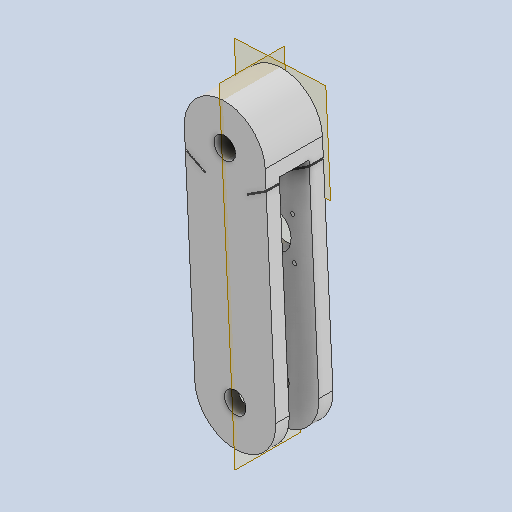
# Autodesk Inventor part: arm segment 2
Saved by Autodesk Inventor 2024 (Build 280153000, 153)
## iProperties
Created: 2024-01-05
Part Number: arm segment 2
Material: Generic
Document SubType Name: Modeling
Designer: MaartenGeorgesBuelen
Density: 1 g/cm^3
Appearance: Default
Author: MaartenGeorgesBuelen
Autodesk Inventor part; units mm, degrees
ref_plane "YZ Plane" through (0, 0, 0) normal (1, 0, 0) x (0, 1, 0)
ref_plane "XZ Plane" through (0, 0, 0) normal (0, 1, 0) x (-1, 0, 0)
ref_plane "Work Plane1" through (-3.789, 77.9897, -50.5078) normal (0, 0, 1) x (0.9988137, 0.0486948, 0)
sketch "Sketch1" plane through (-3.789, 77.9897, -50.5078) normal (0, 0, 1) x (0.9988137, 0.0486948, 0)
  arc A0 (29.7203, 14.7064) -> (-30.2768, 14.1208) centre (-0.263, 12.8566) ccw projected
  circle A1 centre (-0.263, 12.8566) radius 30.0404
  line L0 (25.8606, -3.9877) -> (23.2644, -5.4805)
  line L1 (23.2644, -5.4805) -> (23.0289, -5.0709)
  line L2 (23.0289, -5.0709) -> (23.1978, -4.9738)
  arc A2 (23.1978, -4.9738) -> (23.2457, -4.8334) centre (23.1417, -4.8762) ccw
  arc A3 (23.1909, -4.5987) -> (23.2457, -4.8334) centre (23.9391, -4.5475) ccw
  arc A4 (23.8396, -4.2256) -> (23.1909, -4.5987) centre (23.6062, -4.5703) ccw
  arc A5 (24.0148, -4.3911) -> (23.8396, -4.2256) centre (23.419, -4.8466) ccw
  arc A6 (24.0148, -4.3911) -> (24.1603, -4.4203) centre (24.1042, -4.3228) ccw
  line L3 (24.1603, -4.4203) -> (24.4982, -4.2261)
  arc A7 (24.4982, -4.2261) -> (24.5461, -4.0857) centre (24.4421, -4.1285) ccw
  arc A8 (24.4912, -3.8509) -> (24.5461, -4.0857) centre (25.2395, -3.7998) ccw
  arc A9 (25.1399, -3.4779) -> (24.4912, -3.8509) centre (24.9065, -3.8226) ccw
  arc A10 (25.3152, -3.6434) -> (25.1399, -3.4779) centre (24.7193, -4.0989) ccw
  arc A11 (25.3152, -3.6434) -> (25.4607, -3.6726) centre (25.4046, -3.5751) ccw
  line L4 (25.4607, -3.6726) -> (25.6251, -3.5781)
  line L5 (23.2786, -5.4919) -> (20.6824, -6.9847)
  line L6 (21.5783, -5.9245) -> (21.9162, -5.7302)
  arc A12 (21.9162, -5.7302) -> (21.9641, -5.5898) centre (21.8601, -5.6327) ccw
  arc A13 (21.9092, -5.3551) -> (21.9641, -5.5898) centre (22.6575, -5.304) ccw
  arc A14 (22.5579, -4.9821) -> (21.9092, -5.3551) centre (22.3245, -5.3267) ccw
  arc A15 (22.7332, -5.1476) -> (22.5579, -4.9821) centre (22.1373, -5.6031) ccw
  arc A16 (22.7332, -5.1476) -> (22.8787, -5.1768) centre (22.8226, -5.0793) ccw
  line L7 (22.8787, -5.1768) -> (23.0431, -5.0822)
  line L8 (20.6824, -6.9847) -> (20.4469, -6.5751)
  line L9 (20.4469, -6.5751) -> (20.6158, -6.478)
  arc A17 (21.4328, -5.8953) -> (21.5783, -5.9245) centre (21.5222, -5.827) ccw
  arc A18 (21.4328, -5.8953) -> (21.2576, -5.7298) centre (20.837, -6.3508) ccw
  arc A19 (21.2576, -5.7298) -> (20.6089, -6.1028) centre (21.0242, -6.0744) ccw
  arc A20 (20.6089, -6.1028) -> (20.6637, -6.3375) centre (21.3571, -6.0517) ccw
  arc A21 (20.6158, -6.478) -> (20.6637, -6.3375) centre (20.5597, -6.3804) ccw
  line L10 (20.7516, -6.9254) -> (18.1554, -8.4182)
  line L11 (19.0513, -7.3581) -> (19.3891, -7.1638)
  arc A22 (19.3891, -7.1638) -> (19.4371, -7.0234) centre (19.3331, -7.0663) ccw
  arc A23 (19.3822, -6.7887) -> (19.4371, -7.0234) centre (20.1305, -6.7375) ccw
  arc A24 (20.0309, -6.4156) -> (19.3822, -6.7887) centre (19.7975, -6.7603) ccw
  arc A25 (20.2062, -6.5811) -> (20.0309, -6.4156) centre (19.6103, -7.0366) ccw
  arc A26 (20.2062, -6.5811) -> (20.3516, -6.6103) centre (20.2956, -6.5128) ccw
  line L12 (20.3516, -6.6103) -> (20.5161, -6.5158)
  line L13 (18.1554, -8.4182) -> (17.9199, -8.0086)
  line L14 (17.9199, -8.0086) -> (18.0888, -7.9115)
  arc A27 (18.9058, -7.3289) -> (19.0513, -7.3581) centre (18.9952, -7.2605) ccw
  arc A28 (18.9058, -7.3289) -> (18.7306, -7.1634) centre (18.31, -7.7843) ccw
  arc A29 (18.7306, -7.1634) -> (18.0819, -7.5364) centre (18.4971, -7.508) ccw
  arc A30 (18.0819, -7.5364) -> (18.1367, -7.7711) centre (18.8301, -7.4852) ccw
  arc A31 (18.0888, -7.9115) -> (18.1367, -7.7711) centre (18.0327, -7.814) ccw
  line L15 (18.2037, -8.3904) -> (15.6075, -9.8833)
  line L16 (16.5034, -8.8231) -> (16.8413, -8.6288)
  arc A32 (16.8413, -8.6288) -> (16.8892, -8.4884) centre (16.7852, -8.5313) ccw
  arc A33 (16.8343, -8.2537) -> (16.8892, -8.4884) centre (17.5826, -8.2026) ccw
  arc A34 (17.4831, -7.8807) -> (16.8343, -8.2537) centre (17.2496, -8.2253) ccw
  arc A35 (17.6583, -8.0462) -> (17.4831, -7.8807) centre (17.0625, -8.5016) ccw
  arc A36 (17.6583, -8.0462) -> (17.8038, -8.0754) centre (17.7477, -7.9779) ccw
  line L17 (17.8038, -8.0754) -> (17.9682, -7.9808)
  line L18 (15.6075, -9.8833) -> (15.372, -9.4737)
  line L19 (15.372, -9.4737) -> (15.5409, -9.3765)
  arc A37 (16.358, -8.7939) -> (16.5034, -8.8231) centre (16.4473, -8.7256) ccw
  arc A38 (16.358, -8.7939) -> (16.1827, -8.6284) centre (15.7621, -9.2494) ccw
  arc A39 (16.1827, -8.6284) -> (15.534, -9.0014) centre (15.9493, -8.973) ccw
  arc A40 (15.534, -9.0014) -> (15.5889, -9.2361) centre (16.2822, -8.9503) ccw
  arc A41 (15.5409, -9.3765) -> (15.5889, -9.2361) centre (15.4848, -9.279) ccw
  line L20 (20.5161, -6.5158) -> (20.6588, -6.4337)
  line L21 (20.6506, -6.9835) -> (20.6824, -6.9847)
  line L22 (23.0238, -5.0934) -> (23.0289, -5.0709)
  line L23 (23.2786, -5.4919) -> (23.3153, -5.4513)
  line L24 (-0.263, 12.8566) -> (-0.263, -17.1838)
  line L25 (-26.3867, -3.9877) -> (-23.7905, -5.4805)
  line L26 (-24.6864, -4.4203) -> (-25.0243, -4.2261)
  arc A42 (-25.0722, -4.0857) -> (-25.0243, -4.2261) centre (-24.9682, -4.1285) ccw
  arc A43 (-25.0722, -4.0857) -> (-25.0173, -3.8509) centre (-25.7656, -3.7998) ccw
  arc A44 (-25.0173, -3.8509) -> (-25.666, -3.4779) centre (-25.4326, -3.8226) ccw
  arc A45 (-25.666, -3.4779) -> (-25.8413, -3.6434) centre (-25.2454, -4.0989) ccw
  arc A46 (-25.9867, -3.6726) -> (-25.8413, -3.6434) centre (-25.9307, -3.5751) ccw
  line L27 (-25.9867, -3.6726) -> (-26.1512, -3.5781)
  line L28 (-23.7905, -5.4805) -> (-23.555, -5.0709)
  line L29 (-23.555, -5.0709) -> (-23.7239, -4.9738)
  arc A47 (-24.6864, -4.4203) -> (-24.5409, -4.3911) centre (-24.6303, -4.3228) ccw
  arc A48 (-24.3657, -4.2256) -> (-24.5409, -4.3911) centre (-23.9451, -4.8466) ccw
  arc A49 (-23.717, -4.5987) -> (-24.3657, -4.2256) centre (-24.1322, -4.5703) ccw
  arc A50 (-23.7718, -4.8334) -> (-23.717, -4.5987) centre (-24.4652, -4.5475) ccw
  arc A51 (-23.7718, -4.8334) -> (-23.7239, -4.9738) centre (-23.6678, -4.8762) ccw
  line L30 (-21.2085, -6.9847) -> (-20.973, -6.5751)
  line L31 (-20.973, -6.5751) -> (-21.1419, -6.478)
  arc A52 (-21.1898, -6.3375) -> (-21.1419, -6.478) centre (-21.0858, -6.3804) ccw
  arc A53 (-21.1898, -6.3375) -> (-21.135, -6.1028) centre (-21.8832, -6.0517) ccw
  arc A54 (-22.1044, -5.9245) -> (-21.9589, -5.8953) centre (-22.0483, -5.827) ccw
  arc A55 (-21.135, -6.1028) -> (-21.7837, -5.7298) centre (-21.5502, -6.0744) ccw
  arc A56 (-21.7837, -5.7298) -> (-21.9589, -5.8953) centre (-21.3631, -6.3508) ccw
  line L32 (-23.8047, -5.4919) -> (-21.2085, -6.9847)
  line L33 (-22.1044, -5.9245) -> (-22.4423, -5.7302)
  arc A57 (-22.4902, -5.5898) -> (-22.4423, -5.7302) centre (-22.3862, -5.6327) ccw
  arc A58 (-22.4902, -5.5898) -> (-22.4353, -5.3551) centre (-23.1836, -5.304) ccw
  arc A59 (-22.4353, -5.3551) -> (-23.084, -4.9821) centre (-22.8506, -5.3267) ccw
  arc A60 (-23.4047, -5.1768) -> (-23.2593, -5.1476) centre (-23.3487, -5.0793) ccw
  line L34 (-23.4047, -5.1768) -> (-23.5692, -5.0822)
  arc A61 (-23.084, -4.9821) -> (-23.2593, -5.1476) centre (-22.6634, -5.6031) ccw
  line L35 (-18.6815, -8.4182) -> (-18.4459, -8.0086)
  line L36 (-18.4459, -8.0086) -> (-18.6149, -7.9115)
  arc A62 (-18.6628, -7.7711) -> (-18.6149, -7.9115) centre (-18.5588, -7.814) ccw
  arc A63 (-18.6628, -7.7711) -> (-18.6079, -7.5364) centre (-19.3562, -7.4852) ccw
  arc A64 (-19.5774, -7.3581) -> (-19.4319, -7.3289) centre (-19.5213, -7.2605) ccw
  arc A65 (-18.6079, -7.5364) -> (-19.2567, -7.1634) centre (-19.0232, -7.508) ccw
  arc A66 (-19.2567, -7.1634) -> (-19.4319, -7.3289) centre (-18.836, -7.7843) ccw
  line L37 (-21.2777, -6.9254) -> (-18.6815, -8.4182)
  line L38 (-19.5774, -7.3581) -> (-19.9152, -7.1638)
  arc A67 (-19.9632, -7.0234) -> (-19.9152, -7.1638) centre (-19.8592, -7.0663) ccw
  arc A68 (-19.9632, -7.0234) -> (-19.9083, -6.7887) centre (-20.6565, -6.7375) ccw
  arc A69 (-19.9083, -6.7887) -> (-20.557, -6.4156) centre (-20.3236, -6.7603) ccw
  arc A70 (-20.8777, -6.6103) -> (-20.7323, -6.5811) centre (-20.8216, -6.5128) ccw
  line L39 (-20.8777, -6.6103) -> (-21.0422, -6.5158)
  arc A71 (-20.557, -6.4156) -> (-20.7323, -6.5811) centre (-20.1364, -7.0366) ccw
  line L40 (-16.1336, -9.8833) -> (-15.8981, -9.4737)
  line L41 (-15.8981, -9.4737) -> (-16.067, -9.3765)
  arc A72 (-16.1149, -9.2361) -> (-16.067, -9.3765) centre (-16.0109, -9.279) ccw
  arc A73 (-16.1149, -9.2361) -> (-16.0601, -9.0014) centre (-16.8083, -8.9503) ccw
  arc A74 (-17.0295, -8.8231) -> (-16.884, -8.7939) centre (-16.9734, -8.7256) ccw
  arc A75 (-16.0601, -9.0014) -> (-16.7088, -8.6284) centre (-16.4754, -8.973) ccw
  arc A76 (-16.7088, -8.6284) -> (-16.884, -8.7939) centre (-16.2882, -9.2494) ccw
  line L42 (-18.7298, -8.3904) -> (-16.1336, -9.8833)
  line L43 (-17.0295, -8.8231) -> (-17.3674, -8.6288)
  arc A77 (-17.4153, -8.4884) -> (-17.3674, -8.6288) centre (-17.3113, -8.5313) ccw
  arc A78 (-17.4153, -8.4884) -> (-17.3604, -8.2537) centre (-18.1087, -8.2026) ccw
  arc A79 (-17.3604, -8.2537) -> (-18.0091, -7.8807) centre (-17.7757, -8.2253) ccw
  arc A80 (-18.3299, -8.0754) -> (-18.1844, -8.0462) centre (-18.2738, -7.9779) ccw
  line L44 (-18.3299, -8.0754) -> (-18.4943, -7.9808)
  arc A81 (-18.0091, -7.8807) -> (-18.1844, -8.0462) centre (-17.5885, -8.5016) ccw
  line L45 (-21.0422, -6.5158) -> (-21.1849, -6.4337)
  line L46 (-21.1767, -6.9835) -> (-21.2085, -6.9847)
  line L47 (-23.5499, -5.0934) -> (-23.555, -5.0709)
  line L48 (-23.8047, -5.4919) -> (-23.8414, -5.4513)
  line L49 (-30.3034, 12.8566) -> (29.7773, 12.8566)
  line L50 (29.7773, 12.8566) -> (29.7773, -147.1434)
  line L51 (29.7773, -147.1434) -> (-30.3034, -147.1434)
  line L52 (-30.3034, -147.1434) -> (-30.3034, 12.8566)
  circle A82 centre (-0.263, -147.1434) radius 30.0404
  circle A83 centre (-0.263, -147.1434) radius 8
  line L53 (28.4116, -2.5222) -> (28.176, -2.1125)
  line L54 (25.8637, -3.9872) -> (25.6282, -3.5776)
  line L55 (25.6282, -3.5776) -> (25.7971, -3.4804)
  arc A84 (25.7971, -3.4804) -> (25.845, -3.34) centre (25.741, -3.3829) ccw
  arc A85 (25.7902, -3.1053) -> (25.845, -3.34) centre (26.5384, -3.0542) ccw
  arc A86 (26.6141, -2.8978) -> (26.7596, -2.927) centre (26.7035, -2.8295) ccw
  arc A87 (26.4389, -2.7323) -> (25.7902, -3.1053) centre (26.2055, -3.0769) ccw
  arc A88 (26.6141, -2.8978) -> (26.4389, -2.7323) centre (26.0183, -3.3533) ccw
  line L56 (28.4599, -2.4944) -> (25.8637, -3.9872)
  line L57 (26.7596, -2.927) -> (27.0975, -2.7327)
  arc A89 (27.0975, -2.7327) -> (27.1454, -2.5923) centre (27.0414, -2.6352) ccw
  arc A90 (27.0905, -2.3576) -> (27.1454, -2.5923) centre (27.8388, -2.3065) ccw
  arc A91 (27.7392, -1.9846) -> (27.0905, -2.3576) centre (27.5058, -2.3292) ccw
  arc A92 (27.9145, -2.1501) -> (28.06, -2.1793) centre (28.0039, -2.0818) ccw
  line L58 (28.06, -2.1793) -> (28.2244, -2.0847)
  arc A93 (27.9145, -2.1501) -> (27.7392, -1.9846) centre (27.3186, -2.6056) ccw
  line L59 (28.1819, -2.1049) -> (28.3509, -2.0077)
  line L60 (28.4174, -2.5145) -> (28.1819, -2.1049)
  arc A94 (29.1679, -1.4251) -> (29.3133, -1.4543) centre (29.2573, -1.3568) ccw
  arc A95 (29.6512, -1.26) -> (29.6991, -1.1196) centre (29.5951, -1.1625) ccw
  arc A96 (30.293, -0.5119) -> (29.6443, -0.8849) centre (30.0596, -0.8565) ccw
  line L61 (30.6137, -0.7066) -> (30.7781, -0.612)
  line L62 (30.9653, -1.0494) -> (30.7298, -0.6398)
  arc A97 (30.4682, -0.6774) -> (30.293, -0.5119) centre (29.8724, -1.1328) ccw
  arc A98 (29.6443, -0.8849) -> (29.6991, -1.1196) centre (30.3925, -0.8338) ccw
  arc A99 (28.9926, -1.2596) -> (28.3439, -1.6326) centre (28.7592, -1.6042) ccw
  arc A100 (28.3439, -1.6326) -> (28.3988, -1.8673) centre (29.0922, -1.5815) ccw
  arc A101 (28.3509, -2.0077) -> (28.3988, -1.8673) centre (28.2948, -1.9102) ccw
  arc A102 (29.1679, -1.4251) -> (28.9926, -1.2596) centre (28.572, -1.8806) ccw
  line L63 (31.0137, -1.0216) -> (28.4174, -2.5145)
  arc A103 (30.4682, -0.6774) -> (30.6137, -0.7066) centre (30.5576, -0.6091) ccw
  line L64 (29.3133, -1.4543) -> (29.6512, -1.26)
  line L65 (25.8606, -3.9877) -> (25.8637, -3.9872)
  line L66 (25.6251, -3.5781) -> (25.6282, -3.5776)
  line L67 (-26.1543, -3.5776) -> (-26.3232, -3.4804)
  arc A104 (-27.2857, -2.927) -> (-27.1402, -2.8978) centre (-27.2296, -2.8295) ccw
  arc A105 (-27.6715, -2.5923) -> (-27.6235, -2.7327) centre (-27.5675, -2.6352) ccw
  arc A106 (-27.6166, -2.3576) -> (-28.2653, -1.9846) centre (-28.0319, -2.3292) ccw
  line L68 (-28.586, -2.1793) -> (-28.7505, -2.0847)
  line L69 (-28.9377, -2.5222) -> (-28.7021, -2.1125)
  arc A107 (-28.2653, -1.9846) -> (-28.4406, -2.1501) centre (-27.8447, -2.6056) ccw
  arc A108 (-27.6715, -2.5923) -> (-27.6166, -2.3576) centre (-28.3649, -2.3065) ccw
  arc A109 (-26.3163, -3.1053) -> (-26.965, -2.7323) centre (-26.7315, -3.0769) ccw
  arc A110 (-26.3711, -3.34) -> (-26.3163, -3.1053) centre (-27.0645, -3.0542) ccw
  arc A111 (-26.3711, -3.34) -> (-26.3232, -3.4804) centre (-26.2671, -3.3829) ccw
  arc A112 (-26.965, -2.7323) -> (-27.1402, -2.8978) centre (-26.5444, -3.3533) ccw
  line L70 (-28.986, -2.4944) -> (-26.3898, -3.9872)
  arc A113 (-28.586, -2.1793) -> (-28.4406, -2.1501) centre (-28.53, -2.0818) ccw
  line L71 (-27.2857, -2.927) -> (-27.6235, -2.7327)
  line L72 (-31.4914, -1.0494) -> (-31.2559, -0.6398)
  line L73 (-31.1398, -0.7066) -> (-31.3042, -0.612)
  arc A114 (-31.1398, -0.7066) -> (-30.9943, -0.6774) centre (-31.0837, -0.6091) ccw
  arc A115 (-29.5187, -1.2596) -> (-29.694, -1.4251) centre (-29.0981, -1.8806) ccw
  arc A116 (-30.2252, -1.1196) -> (-30.1773, -1.26) centre (-30.1212, -1.1625) ccw
  arc A117 (-30.2252, -1.1196) -> (-30.1704, -0.8849) centre (-30.9186, -0.8338) ccw
  line L74 (-31.5398, -1.0216) -> (-28.9435, -2.5145)
  arc A118 (-30.1704, -0.8849) -> (-30.8191, -0.5119) centre (-30.5856, -0.8565) ccw
  arc A119 (-30.8191, -0.5119) -> (-30.9943, -0.6774) centre (-30.3985, -1.1328) ccw
  arc A120 (-28.87, -1.6326) -> (-29.5187, -1.2596) centre (-29.2853, -1.6042) ccw
  arc A121 (-28.9249, -1.8673) -> (-28.87, -1.6326) centre (-29.6183, -1.5815) ccw
  arc A122 (-28.9249, -1.8673) -> (-28.8769, -2.0077) centre (-28.8209, -1.9102) ccw
  line L75 (-28.708, -2.1049) -> (-28.8769, -2.0077)
  line L76 (-29.8394, -1.4543) -> (-30.1773, -1.26)
  arc A123 (-29.8394, -1.4543) -> (-29.694, -1.4251) centre (-29.7833, -1.3568) ccw
  line L77 (-28.9435, -2.5145) -> (-28.708, -2.1049)
  line L78 (-26.3867, -3.9877) -> (-26.3898, -3.9872)
  line L79 (-26.1512, -3.5781) -> (-26.1543, -3.5776)
  line L80 (28.4599, -2.4944) -> (28.4581, -2.4911)
  line L81 (-28.9766, -2.4998) -> (-28.9766, -2.4955)
  circle A124 centre (-0.263, 12.8566) radius 8
  point P0 (-0.0132, -78.0817)
  point P1 (29.7507, 11.5924)
  point P2 (23.7394, -5.2074)
  point P3 (20.674, -6.97)
  point P4 (18.1554, -8.4182)
  point P5 (23.0373, -5.0856)
  point P6 (24.4138, -4.2746)
  point P7 (29.7203, 14.7064)
  point P8 (-30.2768, 14.1208)
  point P9 (-24.9399, -4.2746)
  point P10 (-23.5634, -5.0856)
  point P11 (-18.4943, -7.9808)
  point P12 (-21.2001, -6.97)
  point P13 (-24.2654, -5.2074)
  point P14 (24.5453, -4.0836)
  point P15 (-25.0714, -4.0836)
  point P16 (-30.3034, -147.1434)
  point P17 (28.4144, -2.515)
  point P18 (28.1788, -2.1053)
  point P19 (29.7773, -1.7325)
  point P20 (29.7773, -0.5505)
  point P21 (28.176, -2.1125)
  point P22 (28.4116, -2.5222)
  point P23 (-28.9405, -2.515)
  point P24 (-28.7049, -2.1053)
  point P25 (-30.3034, -0.5505)
  point P26 (-30.3034, -1.7325)
  point P27 (-28.9377, -2.5222)
  point P28 (-28.7021, -2.1125)
  point P29 (-28.7099, -2.1081)
  point P30 (28.1838, -2.1081)
  dimension "d2" = 160
  constraints: 246 point on circle, 166 symmetric about line, 164 end point, 124 centre point, 9 point on line, 2 concentric, 2 equal radius, 2 parallel, 2 perpendicular, 1 horizontal, 1 midpoint, 1 vertical, 62 other
  measures "d2" distance of L49.end L50.end
ref_plane "Work Plane2" through (-31.6155, -23.2448, -8) normal (0, 0, -1) x (0.0117226, 0.9999313, 0)
extrude "Extrusion1" add sketch "Sketch1" along normal up to surface (42.5078 mm away) contours A1 L49 A124 A0 | L50 A96 A98 A95 L64 A94 A102 A99 A100 A101 L59 L60 L58 A92 A93 A91 A90 A89 L57 A86 A88 A87 A85 A84 L55 L66 L4 A11 A10 A9 A1 | A1 A9 A8 L3 A6 A5 A4 A3 A2 L2 L22 L7 A16 A15 A14 A13 A12 L6 A17 A18 A19 A20 A21 L20 L12 A26 A25 A24 A23 A22 L11 A27 A28 A29 A30 A31 L14 L17 A36 A35 A34 A33 A32 L16 A37 A38 A39 A40 A41 L19 L18 L15 L10 L21 L5 L23 L0 L24 A124 L49 | L49 A124 L24 A1 L25 L48 L32 L46 L37 L42 L40 L41 A72 A73 A75 A76 A74 L43 A77 A78 A79 A81 A80 L44 L36 A62 A63 A65 A66 A64 L38 A67 A68 A69 A71 A70 L39 L45 A52 A53 A55 A56 A54 L33 A57 A58 A59 A61 A60 L34 L47 L29 A51 A50 A49 A48 A47 L26 A43 A44 | A1 A44 A45 A46 L27 L79 L67 A111 A110 A109 A112 A104 L71 A105 A108 A106 A107 A113 L68 L77 L75 A122 A121 A120 A115 A123 L76 A116 A117 A118 L52 | L50 A82 L52 L74 L81 L70 L78 L25 A1 L0 L65 L56 L80 L63 | A82 L51 A83 | L51 A83 A82 | L7 L22 L1 | L21 L10 L8 | L28 L47 L34 | L30 L37 L46
sketch "Sketch3" plane through (33.1181, -67.5291, -8) normal (0.9988137, 0.0486948, 0) x (0, 0, -1)
  line L0 (0, 0) -> (0, 145.4109) projected
  line L1 (42.0155, 0) -> (0, 0) projected
  line L2 (42.0155, 0) -> (42.0155, 145.4109) projected
  line L3 (42.5078, 160) -> (0, 160) projected
  line L4 (32.0155, 150) -> (32.0155, 10)
  line L5 (32.0155, 10) -> (10, 10)
  line L6 (10, 10) -> (10, 150)
  line L7 (10, 150) -> (32.0155, 150)
  line L8 (0, 146.5929) -> (0, 160) projected
  line L9 (42.5078, 146.5929) -> (0, 146.5929) projected
  line L10 (42.5078, 146.5929) -> (42.5078, 160) projected
  line L11 (42.0155, 145.4109) -> (0, 145.4109) projected
  point P0 (-8, 69.0617)
  dimension "d3" = 10
  constraints: 8 end point, 3 other
  measures "d3" distance between parallel lines of L2 L4
extrude "Extrusion2" cut sketch "Sketch3" against normal through all contours L11 L4 L5 L6 | L6 L9 L4 L11 | L6 L7 L4 L9
ref_plane "Work Plane3" through (3.1134, -68.992, -8) normal (0.9988137, 0.0486948, 0) x (0, 0, -1)
sketch "Sketch4" plane through (32.6312, -57.541, -40.0155) normal (0, 0, 1) x (0.9988137, 0.0486948, 0)
  line L0 (-48.7216, 63.3532) -> (-50.7216, 65.3529) projected
  line L1 (-48.7216, 63.3532) -> (-10.7216, 63.3532) projected
  line L2 (-8.7216, 65.3529) -> (-10.7216, 63.3532) projected
  line L3 (-8.7216, 65.3529) -> (-8.7216, 103.3472) projected
  line L4 (-10.7216, 105.3469) -> (-8.7216, 103.3472) projected
  line L5 (-10.7216, 105.3469) -> (-48.7216, 105.3469) projected
  line L6 (-50.7216, 103.3472) -> (-48.7216, 105.3469) projected
  line L7 (-50.7216, 103.3472) -> (-50.7216, 65.3529) projected
  circle A0 centre (-30, 84) radius 14
  ellipse E0 centre (-14.2216, 68.8524) end of major axis (-12.7216, 68.8524) minor radius 1.4998 projected
  ellipse E1 centre (-14.2216, 99.8478) end of major axis (-12.7216, 99.8478) minor radius 1.4998 projected
  ellipse E2 centre (-45.2216, 68.8524) end of major axis (-43.7216, 68.8524) minor radius 1.4998 projected
  ellipse E3 centre (-45.2216, 99.8478) end of major axis (-43.7216, 99.8478) minor radius 1.4998 projected
  ellipse E4 centre (-29.7216, 84.3501) end of major axis (-18.7216, 84.3501) minor radius 10.9984 projected
  point P0 (-29.7905, 59.0617)
  constraints: 1 centre point
extrude "Extrusion3" cut sketch "Sketch4" against normal through all contours A0 | E0 | E1 | E2 | E3 | E4
sketch "Sketch6" plane through (32.6312, -57.541, -40.0155) normal (0, 0, 1) x (0.9988137, 0.0486948, 0)
  line L0 (0, 0) -> (-60.0808, 0) projected
  arc A0 (-60.0808, -10) -> (0, -10) centre (-30.0404, -10) ccw projected
  line L1 (0, -10) -> (0, 150) projected
  line L2 (-60.0808, 150) -> (-60.0808, -10) projected
  point P0 (-29.7905, 59.0617)
extrude "Extrusion4" cut sketch "Sketch6" along normal up to surface (22.0155 mm away)
body "Solid1"
